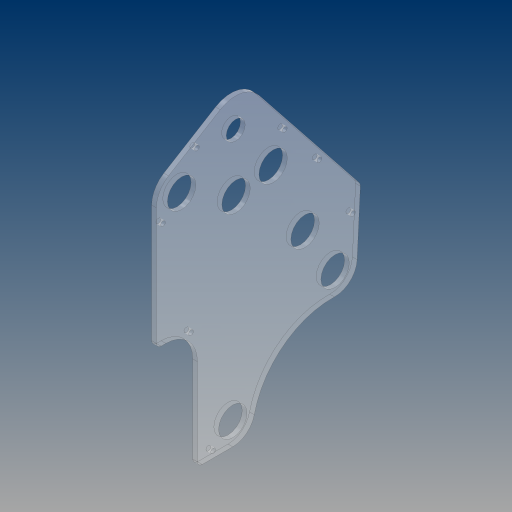
# Autodesk Inventor part: INTK_001_PulleyCover
Saved by Autodesk Inventor 2024.3 (Build 283343000, 343)
## iProperties
Created: 2024-08-04
Part Number: INTK_001_PulleyCover
Material: Polycarbonate, Clear
Document SubType Name: Modeling
Designer: Kenji
Density: 1.2 g/cm^3
Appearance: Polycarbonate - Clear
Author: Kenji
Autodesk Inventor part; units mm, degrees
ref_plane "YZ Plane" through (0, 0, 0) normal (1, 0, 0) x (0, 1, 0)
ref_plane "XZ Plane" through (0, 0, 0) normal (0, 1, 0) x (-1, 0, 0)
ref_plane "XY Plane" through (0, 0, 0) normal (0, 0, 1) x (1, 0, 0)
sketch "Sketch1" plane through (0, 0, 0) normal (1, 0, 0) x (0, 1, 0)
  line L0 (95.25, -63.5) -> (7.9502, -63.5) construction
  arc A0 (95.25, -63.5) -> (127, -31.75) centre (95.25, -31.75) ccw construction
  circle A1 centre (104.9083, -202.0677) radius 25.4 construction
  circle A2 centre (104.9083, -202.0677) radius 14.2875
  circle A3 centre (154.8209, -171.8196) radius 25.4 construction
  circle A4 centre (154.8209, -171.8196) radius 14.2875
  circle A5 centre (250.0002, -47.5843) radius 22.225 construction
  circle A6 centre (250.0002, -47.5843) radius 25.4 construction
  circle A7 centre (250.0002, -47.5843) radius 14.2875
  circle A8 centre (154.8209, -171.8196) radius 22.225 construction
  circle A9 centre (104.9083, -202.0677) radius 22.225 construction
  circle A10 centre (25.4, -99.06) radius 25.4 construction
  circle A11 centre (25.4, -99.06) radius 23.8125 construction
  line L1 (25.4, -73.66) -> (25.4, -63.5) construction
  circle A12 centre (219.8086, -102.3786) radius 25.4 construction
  circle A13 centre (219.8086, -102.3786) radius 22.225 construction
  circle A14 centre (219.8086, -102.3786) radius 14.2875
  circle A15 centre (63.172, -79.375) radius 6.477 construction
  circle A16 centre (25.4, -99.06) radius 14.2875
  circle A17 centre (63.172, -79.375) radius 3.2512 construction
  circle A18 centre (166.1747, -221.0415) radius 3.2512 construction
  line L2 (219.8086, -102.3786) -> (154.8209, -171.8196) construction
  line L3 (154.8209, -171.8196) -> (104.9083, -202.0677) construction
  circle A19 centre (166.1747, -221.0415) radius 6.4262 construction
  circle A20 centre (63.172, -79.375) radius 6.35 construction
  circle A21 centre (25.4, -99.06) radius 22.225 construction
  line L4 (3.175, -99.06) -> (3.175, -68.2752)
  arc A22 (166.1747, -227.4677) -> (170.1786, -226.0679) centre (166.1747, -221.0415) ccw
  arc A23 (3.175, -99.06) -> (20.3984, -120.7149) centre (25.4, -99.06) ccw
  arc A24 (7.9502, -63.5) -> (3.175, -68.2752) centre (7.9502, -68.2752) ccw
  line L5 (232.868, -28.832) -> (267.1324, -66.3365) construction
  circle A25 centre (232.868, -28.832) radius 2.4257
  circle A26 centre (267.1324, -66.3365) radius 2.4257 construction
  circle A27 centre (232.868, -28.832) radius 6.35 construction
  circle A28 centre (267.1324, -66.3365) radius 6.35 construction
  line L6 (219.8086, -102.3786) -> (237.1646, -83.8332) construction
  line L7 (219.8086, -102.3786) -> (202.4526, -120.9239) construction
  circle A29 centre (237.1646, -83.8332) radius 2.4257 construction
  circle A30 centre (202.4526, -120.9239) radius 2.4257 construction
  circle A31 centre (172.1769, -153.2743) radius 2.4257 construction
  circle A32 centre (133.0985, -184.9838) radius 2.4257 construction
  arc A33 (82.6927, -201.4208) -> (103.7686, -224.2634) centre (104.9083, -202.0677) ccw
  circle A34 centre (9.525, -79.2321) radius 2.4257
  circle A35 centre (9.525, -79.2321) radius 6.35 construction
  arc A36 (82.6927, -201.4208) -> (20.3984, -120.7149) centre (2.2987, -199.0799) ccw
  line L8 (9.525, -79.2321) -> (41.275, -118.8879) construction
  circle A37 centre (41.275, -118.8879) radius 2.4257 construction
  circle A38 centre (41.275, -118.8879) radius 5.6007 construction
  line L9 (7.9502, -63.5) -> (95.25, -63.5)
  arc A39 (95.25, -63.5) -> (127, -31.75) centre (95.25, -31.75) ccw
  line L10 (166.1747, -227.4677) -> (103.7686, -224.2634)
  line L11 (104.9083, -202.0677) -> (83.1859, -215.2319) construction
  line L12 (127, -31.75) -> (127, -26.9595)
  circle A40 centre (133.0985, -184.9838) radius 5.6007 construction
  circle A41 centre (277.7476, -102.0288) radius 30 construction
  circle A42 centre (277.7476, -102.0288) radius 25.4 construction
  circle A43 centre (277.7476, -102.0288) radius 9.525
  circle A44 centre (219.8086, -102.3786) radius 19.05 construction
  circle A45 centre (227.4601, -139.7023) radius 19.05 construction
  circle A46 centre (227.4601, -139.7023) radius 14.2875
  line L13 (247.7482, -102.2099) -> (245.2082, -102.2252) construction
  line L14 (170.1786, -226.0679) -> (296.4391, -125.4942)
  arc A47 (296.4391, -125.4942) -> (303.3752, -86.4331) centre (277.7476, -102.0288) ccw
  circle A48 centre (219.8086, -102.3786) radius 30.48 construction
  circle A49 centre (277.7476, -102.0288) radius 30.48 construction
  circle A50 centre (248.6408, -79.4624) radius 3.81 construction
  line L15 (251.6519, -81.7968) -> (253.6592, -83.3531) construction
  line L16 (245.6582, -81.833) -> (243.6698, -83.4134) construction
  circle A51 centre (248.6408, -79.4624) radius 2.3812 construction
  circle A52 centre (248.9154, -124.945) radius 3.81 construction
  circle A53 centre (248.9154, -124.945) radius 2.3876 construction
  line L17 (251.898, -122.5744) -> (253.8865, -120.9939) construction
  line L18 (245.9043, -122.6105) -> (243.897, -121.0542) construction
  line L19 (248.6408, -75.6524) -> (248.6408, -72.9479) construction
  line L20 (219.8086, -102.3786) -> (219.8086, -88.0911) construction
  line L21 (131.7752, -22.1843) -> (250.0002, -22.1843)
  line L22 (271.6983, -34.3799) -> (303.3752, -86.4331)
  arc A54 (271.6983, -34.3799) -> (250.0002, -22.1843) centre (250.0002, -47.5843) ccw
  arc A55 (131.7752, -22.1843) -> (127, -26.9595) centre (131.7752, -26.9595) ccw
  circle A56 centre (146.08, -220.0775) radius 6.35 construction
  circle A57 centre (146.08, -220.0775) radius 2.4257
  circle A58 centre (253.6387, -151.4689) radius 6.35 construction
  circle A59 centre (253.6387, -151.4689) radius 2.4257
  circle A60 centre (209.9304, -186.285) radius 6.35 construction
  circle A61 centre (209.9304, -186.285) radius 2.4257
  circle A62 centre (123.7263, -57.0623) radius 6.35 construction
  circle A63 centre (123.7263, -57.0623) radius 2.4257
  circle A64 centre (281.6771, -62.9926) radius 6.35 construction
  circle A65 centre (281.6771, -62.9926) radius 2.4257
  line L23 (123.7263, -57.0623) -> (232.868, -28.832) construction
  line L24 (232.868, -28.832) -> (281.6771, -62.9926) construction
  line L25 (281.6771, -62.9926) -> (253.6387, -151.4689) construction
  line L26 (253.6387, -151.4689) -> (209.9304, -186.285) construction
  line L27 (209.9304, -186.285) -> (146.08, -220.0775) construction
  line L28 (146.08, -220.0775) -> (9.525, -79.2321) construction
  line L29 (123.7263, -57.0623) -> (9.525, -79.2321) construction
  point P0 (180.2209, -171.8196)
  point P1 (172.6009, -221.0415)
  point P2 (104.9083, -227.4677)
  point P3 (127, -22.1843)
  point P4 (250.0002, -47.5843)
  point P5 (0, 0)
  point P6 (95.25, -63.5)
  dimension "d4" = 31.75
  dimension "d17" = 50.8
  dimension "d18" = 1.5875
  dimension "d21" = 12.954
  dimension "d22" = 28.575
  dimension "d23" = 6.5024
  dimension "d26" = 130.175
  dimension "d27" = 15.875
  dimension "d28" = 6.5024
  dimension "d29" = 143.1895
  dimension "d41" = 3.175
  dimension "d42" = 12.7
  dimension "d43" = 10.16
  dimension "d44" = 50.8
  dimension "d45" = 3.175
  dimension "d46" = 44.45
  dimension "d53" = 3.175
  dimension "d55" = 4.7752
  dimension "d59" = 4.8514
  dimension "d60" = 4.8514
  dimension "d68" = 4.8514
  dimension "d69" = 4.8514
  dimension "d70" = 4.8514
  dimension "d71" = 4.8514
  dimension "d72" = 4.8514
  dimension "d74" = 4.8514
  dimension "d75" = 3.175
  dimension "d86" = 7.62
  dimension "d88" = 3.175
  dimension "d90" = 58.3628
  dimension "d92" = 60
  dimension "d93" = 50.8
  dimension "d96" = 19.05
  dimension "d97" = 38.1
  dimension "d98" = 38.1
  dimension "d99" = 28.575
  dimension "d100" = 56.9248
  dimension "d101" = 2.54
  dimension "d102" = 60.96
  dimension "d103" = 60.96
  dimension "d104" = 7.62
  dimension "d105" = 2.54
  dimension "d106" = 4.7625
  dimension "d107" = 7.62
  dimension "d108" = 4.7752
  dimension "d109" = 2.54
  dimension "d111" = 2.7045
  dimension "d112" = 38.682
  dimension "d113" = 7.6515
  dimension "d114" = 202.0601
  dimension "d115" = 40.6423
  dimension "d116" = 37.3238
  dimension "d117" = 95.1077
  dimension "d118" = 57.939
  dimension "d119" = 62.8341
  dimension "d120" = 61.1075
  dimension "d121" = 250.0002
  dimension "d122" = 99.06
  dimension "d123" = 25.4
  dimension "d125" = 127
  dimension "d127" = 80.428
  dimension "d128" = 130.1236
  dimension "d129" = 232.868
  dimension "d130" = 4.7752
  constraints: 65 centre point, 60 end point, 55 point on circle, 24 coincident, 21 tangent, 18 point on line, 11 concentric, 9 equal radius, 4 midpoint, 4 vertical, 3 collinear, 3 horizontal alignment, 3 vertical alignment, 2 equal length, 2 horizontal, 1 perpendicular, 5 other
  measures "d4" radius of A0
  measures "d17" diameter of A10
  measures "d18" radial gap between concentric circles of A10 A11
  measures "d21" diameter of A15
  measures "d22" diameter of A16
  measures "d23" diameter of A17
  measures "d26" distance of A15.centre A8.centre
  measures "d27" distance from line of L0 A15.centre
  measures "d28" diameter of A18
  measures "d29" distance of A0.centre A13.centre
  measures "d41" radial gap between concentric circles of A18 A19
  measures "d42" diameter of A20
  measures "d43" distance of L1.start L1.end
  measures "d44" diameter of A3
  measures "d45" radial gap between concentric circles of A9 A1
  measures "d46" diameter of A9
  measures "d53" radial gap between concentric circles of A10 A21
  measures "d55" radius of A24
  measures "d59" diameter of A25
  measures "d60" diameter of A26
  measures "d68" diameter of A29
  measures "d69" diameter of A30
  measures "d70" diameter of A31
  measures "d71" diameter of A32
  measures "d72" diameter of A34
  measures "d74" diameter of A37
  measures "d75" radial gap between concentric circles of A37 A38
  measures "d86" horizontal distance of A19.start A3.start
  measures "d88" radial gap between concentric circles of A32 A40
  measures "d90" distance of L2.end L3.end
  measures "d92" diameter of A41
  measures "d93" diameter of A42
  measures "d96" diameter of A43
  measures "d97" diameter of A44
  measures "d98" diameter of A45
  measures "d99" diameter of A46
  measures "d100" distance of A31.centre A45.centre
  measures "d101" horizontal distance of L13.start L13.end
  measures "d102" diameter of A48
  measures "d103" diameter of A49
  measures "d104" diameter of A50
  measures "d105" distance of L15.start L15.end
  measures "d106" diameter of A51
  measures "d107" diameter of A52
  measures "d108" diameter of A53
  measures "d109" distance of L17.start L17.end
  measures "d111" distance of L19.start L19.end
  measures "d112" angle of L8 L1
  measures "d113" horizontal distance of A44.centre A45.centre
  measures "d114" horizontal distance of A45.centre point (25.4, -99.06)
  measures "d115" vertical distance of A45.centre A16.centre
  measures "d116" vertical distance of A13.centre A45.centre
  measures "d117" distance of L6.start L2.end
  measures "d118" horizontal distance of L20.start A41.centre
  measures "d119" distance of A45.centre A41.centre
  measures "d120" distance of A5.centre A41.centre
  measures "d121" horizontal distance of point (0, 0) A5.centre
  measures "d122" vertical distance of A11.centre point (0, 0)
  measures "d123" horizontal distance of A11.centre point (0, 0)
  measures "d125" distance from line of point (0, 0) L12
  measures "d127" radius of A36
  measures "d128" distance of A16.centre A9.centre
  measures "d129" horizontal distance of point (0, 0) L5.start
  measures "d130" radius of A55
extrude "Extrusion1" add sketch "Sketch1" along normal blind 4.7625
body "Solid1"
